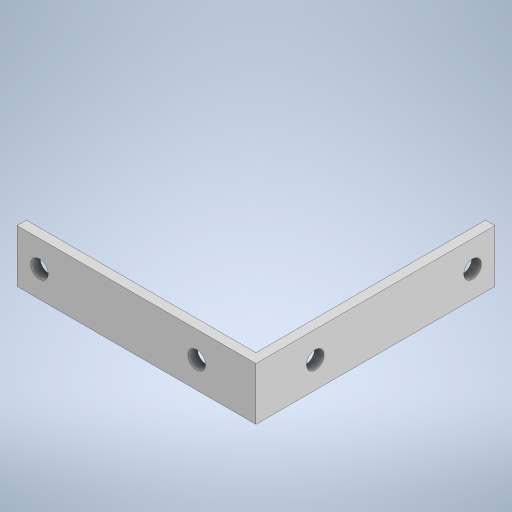
# Autodesk Inventor part: Lbracket
Saved by Autodesk Inventor 2024.3 (Build 283343000, 343)
## iProperties
Created: 2024-11-20
Part Number: Lbracket
Material: Generic
Document SubType Name: Modeling
Designer: email
Density: 1 g/cm^3
Appearance: Default
Author: email
Autodesk Inventor part; units mm, degrees
ref_plane "YZ Plane" through (0, 0, 0) normal (1, 0, 0) x (0, 1, 0)
ref_plane "XZ Plane" through (0, 0, 0) normal (0, 1, 0) x (-1, 0, 0)
ref_plane "XY Plane" through (0, 0, 0) normal (0, 0, 1) x (1, 0, 0)
sketch "Sketch1" plane through (0, 0, 0) normal (0, 1, 0) x (-1, 0, 0)
  line L0 (0, 0) -> (-102, 0)
  line L1 (-102, 0) -> (-102, -4)
  line L2 (-102, -4) -> (0, -4)
  line L3 (0, -4) -> (0, 0)
  line L4 (-102, 0) -> (-98, 0)
  line L5 (-98, 0) -> (-98, -102)
  line L6 (-98, -102) -> (-102, -102)
  line L7 (-102, -102) -> (-102, 0)
  point P0 (-98, -4)
  dimension "d0" = 102
  dimension "d1" = 4
  dimension "d2" = 102
  dimension "d3" = 4
  constraints: 16 end point, 4 parallel, 2 horizontal, 2 perpendicular
  measures "d0" distance of L0.start L0.end
  measures "d1" distance of L2.end L0.start
  measures "d2" distance of L6.end L0.end
  measures "d3" distance of L5.end L6.end
extrude "Extrusion1" add sketch "Sketch1" along normal blind 22.5
sketch "Sketch2" plane through (102, 0, 0) normal (1, 0, 0) x (0, 0, -1)
  line L0 (102, 0) -> (102, 22.5) projected
  line L1 (102, 11.25) -> (96, 11.25) construction
  circle A0 centre (92.425, 11.25) radius 3.575
  line L2 (88.85, 11.25) -> (28.85, 11.25) construction
  circle A1 centre (25.275, 11.25) radius 3.575
  line L3 (0, 0) -> (0, 22.5) projected
  line L4 (0, 22.5) -> (102, 22.5) projected
  point P0 (0, 11.25)
  dimension "d9" = 7.15
  dimension "d6" = 6
  dimension "d7" = 7.15
  dimension "d8" = 60
  dimension "d29" = 25.275
  dimension "d30" = 11.25
  constraints: 4 end point, 2 horizontal, 2 midpoint, 2 point on circle, 1 centre point, 1 horizontal alignment, 2 other
  measures "d6" distance of L1.start L1.end
  measures "d7" diameter of A0
  measures "d8" distance of L2.start L2.end
  measures "d29" distance of point (0, 11.25) point (25.275, 11.25)
  measures "d30" distance from line of L4 point (25.275, 11.25)
sketch "Sketch3" plane through (0, 0, 0) normal (0, 0, 1) x (1, 0, 0)
  line L0 (102, 0) -> (102, 22.5) projected
  circle A0 centre (76.725, 11.25) radius 3.575
  line L1 (73.15, 11.25) -> (13.15, 11.25)
  circle A1 centre (9.575, 11.25) radius 3.575
  line L2 (0, 11.25) -> (6, 11.25)
  point P0 (0, 0)
  dimension "d11" = 7.15
  dimension "d12" = 60
  dimension "d13" = 7.15
  dimension "d28" = 6
  constraints: 4 end point, 2 horizontal, 2 point on circle, 1 centre point, 1 horizontal alignment, 2 other
  measures "d12" distance of L1.start L1.end
  measures "d13" diameter of A1
  measures "d28" distance of L2.start L2.end
hole "Hole1" at (102, 11.25, -92.425) at (102, 11.25, -25.275) direction (-1, 0, 0) diameter 7.5 depth 10
hole "Hole2" at (9.575, 11.25, 0) at (76.725, 11.25, 0) direction (0, 0, -1) diameter 7.5 depth 10
body "Solid1"
